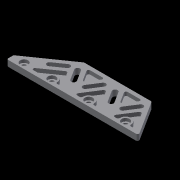
# Autodesk Inventor part: ForearmUpperShockPlate
Saved by Autodesk Inventor 2015 (Build 190159000, 159)
## iProperties
Created: 2014-10-10
Part Number: ForearmUpperShockPlate
Material: Generic
Document SubType Name: Modeling
Designer: Val
Density: 1 g/cm^3
Appearance: Default
Mass: 38.0558 g
Surface Area: 197.178 cm^2
Volume: 38.0558 cm^3
Author: Val
Autodesk Inventor part; units mm, degrees
ref_plane "YZ Plane" through (0, 0, 0) normal (1, 0, 0) x (0, 1, 0)
ref_plane "XZ Plane" through (0, 0, 0) normal (0, 1, 0) x (-1, 0, 0)
ref_plane "XY Plane" through (0, 0, 0) normal (0, 0, 1) x (1, 0, 0)
sketch "Base" plane through (0, 0, 0) normal (0, 0, 1) x (1, 0, 0)
  line L0 (-45.7522, 47.5316) -> (-101, 9)
  line L1 (44.2478, 47.5316) -> (-45.7522, 47.5316)
  line L2 (-48, 0) -> (-101, 0)
  line L3 (0, 0) -> (-48, 0)
  line L4 (49, 0) -> (0, 0)
  line L5 (74.5, 0) -> (44.2478, 47.5316)
  line L6 (49, 0) -> (74.5, 0)
  line L7 (-101, 0) -> (-101, 9)
  dimension "d29" = 16.3728
  dimension "d30" = 16.3728
  dimension "d48" = 57.525
  dimension "d50" = 145.107
  dimension "d51" = 90
  dimension "d52" = 175.5
  dimension "d53" = 9
  dimension "d57" = 53
  dimension "d58" = 48
  dimension "d59" = 49
  constraints: 16 end point, 2 collinear, 1 coincident, 1 horizontal, 1 parallel, 1 perpendicular, 1 point on line
  measures "d48" angle of L5 L6
  measures "d50" angle of L1 L0
  measures "d51" distance of L1.start L1.end
  measures "d52" distance of L5.start L7.start
  measures "d53" distance of L7.start L0.end
  measures "d57" distance of L3.end L7.start
  measures "d58" distance of L4.end L3.end
  measures "d59" distance of L4.start L4.end
extrude "BaseFeature" add sketch "Base" against normal blind 8
fillet "BaseFilletsFeature" radius 2 5 edges at (-101, 9, -4) (-101, 0, -4) (-45.7522, 47.5316, -4) (44.2478, 47.5316, -4) (74.5, 0, -4)
sketch "Sinks" plane through (0, 0, 0) normal (0, 0, 1) x (1, 0, 0)
  line L0 (33.6091, 5) -> (42.4289, 5)
  line L1 (17.2364, 5) -> (7.5711, 5)
  line L2 (17.2364, 5) -> (0.5, 31.2958)
  line L3 (33.6091, 5) -> (49.5, 29.9673)
  line L4 (-32.6091, 5) -> (-41.4289, 5)
  circle A0 centre (0.5, 7.5) radius 7.5
  line L5 (-16.2364, 5) -> (0.5, 31.2958)
  line L6 (-6.5711, 5) -> (-16.2364, 5)
  line L7 (-32.6091, 5) -> (-46.2615, 26.4503)
  circle A1 centre (-85.5, 7.5) radius 7.5
  line L8 (-55.5711, 5) -> (-77.0175, 5)
  line L9 (-46.2615, 26.4503) -> (-77.0175, 5)
  circle A2 centre (-48.5, 7.5) radius 7.5 construction
  line L10 (65.3909, 5) -> (56.5711, 5)
  line L11 (65.3909, 5) -> (49.5, 29.9673)
  circle A3 centre (49.5, 7.5) radius 7.5
  line L12 (37.3455, 42.5316) -> (25.4228, 23.7988)
  line L13 (-12.5, 42.5316) -> (-36.3455, 42.5316)
  line L14 (-24.4228, 23.7988) -> (-12.5, 42.5316)
  line L15 (-24.4228, 23.7988) -> (-36.3455, 42.5316)
  line L16 (13.5, 42.5316) -> (25.4228, 23.7988)
  arc A4 (-41.4289, 5) -> (-55.5711, 5) centre (-48.5, 7.5) ccw
  line L17 (70.8563, 0) -> (-99, 0) construction
  line L18 (-101, 2) -> (-101, 7.9565) projected
  line L19 (44.8372, 46.6055) -> (72.5436, 3.0739) construction
  line L20 (13.5, 42.5316) -> (37.3455, 42.5316)
  line L21 (-45.1237, 47.5316) -> (43.15, 47.5316) construction
  line L22 (-100.1441, 9.5969) -> (-46.2678, 47.172) construction
  line L23 (0.5, 31.2958) -> (0.5, 7.5) construction
  line L24 (49.5, 29.9673) -> (49.5, 7.5) construction
  point P0 (0, 0)
  point P1 (49.5, 0)
  dimension "d17" = 15
  dimension "d18" = 15.5
  dimension "d19" = 37
  dimension "d20" = 49
  dimension "d21" = 49
  dimension "d22" = 5
  dimension "d23" = 5
  dimension "d24" = 5
  dimension "d25" = 17
  dimension "d26" = 17
  dimension "d27" = 17
  dimension "d28" = 17
  dimension "d29" = 16.3728
  dimension "d30" = 16.3728
  dimension "d32" = 26
  dimension "d33" = 0
  dimension "d35" = 17
  constraints: 40 end point, 17 parallel, 9 point on circle, 8 collinear, 5 centre point, 4 tangent, 3 equal radius, 1 concentric, 1 perpendicular, 1 vertical
  measures "d17" diameter of A2
  measures "d18" distance from line of A1.centre L18
  measures "d19" distance of A2.centre A1.centre
  measures "d20" distance of L23.end A2.centre
  measures "d21" distance of L24.end L23.end
  measures "d22" distance between parallel lines of L21 L20
  measures "d23" distance between parallel lines of L19 L11
  measures "d24" distance between parallel lines of L17 L10
  measures "d25" distance between parallel lines of L12 L3
  measures "d26" distance between parallel lines of L2 L16
  measures "d27" distance between parallel lines of L5 L14
  measures "d28" distance between parallel lines of L7 L15
  measures "d29" distance of L3.start L2.start
  measures "d30" distance of L5.start L4.start
  measures "d32" distance of L16.start L13.start
  measures "d33" distance from line of A3.start L17
  measures "d35" distance between parallel lines of L22 L9
extrude "SinksFeature" cut sketch "Sinks" against normal blind 5 contours L3 L11 L10 A3 L0 | L1 A0 L6 L5 L2 | L4 A4 L8 L9 L7 | L12 L16 L20 | L14 L15 L13
fillet "SinkFilletsFeature" radius 2 21 edges at (-46.2615, 26.4503, -2.5) (-77.0175, 5, -2.5) (-32.6091, 5, -2.5) (-55.5711, 5, -2.5) (-41.4289, 5, -2.5) (-36.3455, 42.5316, -2.5) (-12.5, 42.5316, -2.5) (-24.4228, 23.7988, -2.5) (0.5, 31.2958, -2.5) (-16.2364, 5, -2.5) (17.2364, 5, -2.5) (13.5, 42.5316, -2.5) (37.3455, 42.5316, -2.5) (25.4228, 23.7988, -2.5) (49.5, 29.9673, -2.5) (33.6091, 5, -2.5) (65.3909, 5, -2.5) (42.4289, 5, -2.5) (-6.5711, 5, -2.5) (7.5711, 5, -2.5) (56.5711, 5, -2.5)
sketch "Rails" plane through (0, 0, 0) normal (0, 0, 1) x (1, 0, 0)
  line L0 (15.0232, 18.255) -> (5.6268, 33.0184)
  arc A0 (15.0232, 18.255) -> (20.5068, 21.745) centre (17.765, 20) ccw
  line L1 (39.7351, 36.5084) -> (30.3388, 21.745)
  line L2 (35.8223, 18.255) -> (45.2187, 33.0184)
  arc A1 (30.3388, 21.745) -> (35.8223, 18.255) centre (33.0805, 20) ccw
  line L3 (11.1104, 36.5084) -> (20.5068, 21.745)
  arc A2 (45.2187, 33.0184) -> (39.7351, 36.5084) centre (42.4769, 34.7634) ccw
  line L4 (-34.8223, 18.255) -> (-44.2187, 33.0184)
  line L5 (-38.7351, 36.5084) -> (-29.3388, 21.745)
  arc A3 (-34.8223, 18.255) -> (-29.3388, 21.745) centre (-32.0805, 20) ccw
  arc A4 (-38.7351, 36.5084) -> (-44.2187, 33.0184) centre (-41.4769, 34.7634) ccw
  arc A5 (-4.6268, 33.0184) -> (-10.1104, 36.5084) centre (-7.3686, 34.7634) ccw
  line L6 (-14.0232, 18.255) -> (-4.6268, 33.0184)
  line L7 (-10.1104, 36.5084) -> (-19.5068, 21.745)
  arc A6 (-19.5068, 21.745) -> (-14.0232, 18.255) centre (-16.765, 20) ccw
  arc A7 (11.1104, 36.5084) -> (5.6268, 33.0184) centre (8.3686, 34.7634) ccw
  line L8 (-64.9716, 19.8019) -> (-50.6178, 29.8128)
  line L9 (-54.3361, 35.1442) -> (-68.6899, 25.1334)
  arc A8 (-68.6899, 25.1334) -> (-64.9716, 19.8019) centre (-66.8308, 22.4677) ccw
  arc A9 (-50.6178, 29.8128) -> (-54.3361, 35.1442) centre (-52.4769, 32.4785) ccw
  line L10 (-100.1441, 9.5969) -> (-46.2678, 47.172) construction
  line L11 (-71.7978, 8.6404) -> (-47.9727, 25.2568) construction
  line L12 (-45.1413, 24.6903) -> (-34.5656, 8.0739) construction
  line L13 (-26.11, 26.4498) -> (-34.3891, 39.4577) construction
  line L14 (-14.4564, 39.4577) -> (-22.7355, 26.4498) construction
  line L15 (-14.28, 8.0739) -> (-1.1872, 28.6449) construction
  line L16 (2.1872, 28.6449) -> (15.28, 8.0739) construction
  line L17 (23.7355, 26.4498) -> (15.4564, 39.4577) construction
  line L18 (35.3891, 39.4577) -> (27.11, 26.4498) construction
  line L19 (35.5656, 8.0739) -> (47.8128, 27.3164) construction
  line L20 (-32.0805, 20) -> (-16.765, 20) construction
  line L21 (17.765, 20) -> (33.0805, 20) construction
  line L22 (70.8563, 0) -> (-99, 0) construction
  point P0 (0, 0)
  dimension "d29" = 16.3728
  dimension "d30" = 16.3728
  dimension "d36" = 3.25
  dimension "d37" = 17.5
  dimension "d38" = 17
  dimension "d39" = 5.25
  dimension "d40" = 5.25
  dimension "d41" = 5.25
  dimension "d42" = 5.25
  dimension "d43" = 5.25
  dimension "d44" = 5.25
  dimension "d45" = 20
  dimension "d46" = 11
  constraints: 24 end point, 20 point on circle, 10 centre point, 10 equal length, 10 parallel, 9 equal radius, 8 tangent, 2 horizontal
  measures "d36" radius of A9
  measures "d37" distance of L9.start L9.end
  measures "d38" distance between parallel lines of L11 L10
  measures "d39" distance between parallel lines of L11 L8
  measures "d40" distance between parallel lines of L4 L12
  measures "d41" distance between parallel lines of L13 L5
  measures "d42" distance between parallel lines of L14 L7
  measures "d43" distance between parallel lines of L17 L3
  measures "d44" distance between parallel lines of L18 L1
  measures "d45" distance between parallel lines of L22 L21
  measures "d46" horizontal distance of A9.centre A4.centre
extrude "RailsFeature" cut sketch "Rails" against normal through all
hole "BaseHolesFeature" at (-85.5, 7.5, 0) at (-48.5, 7.5, 0) at (0.5, 7.5, 0) at (49.5, 7.5, 0) direction (0, 0, -1) diameter 6 end through all counterbore diameter 10.5 counterbore depth 4
equation "\"d30\" = d29"
equation "\"d23\" = d22"
equation "\"d24\" = d22"
equation "\"d26\" = d25"
equation "\"d27\" = d25"
equation "\"d28\" = d25"
equation "\"d35\" = d25"
equation "\"d39\" = -d36 + 0.5 * d38"
equation "\"d40\" = d39"
equation "\"d41\" = d39"
equation "\"d42\" = d39"
equation "\"d43\" = d39"
equation "\"d44\" = d39"
